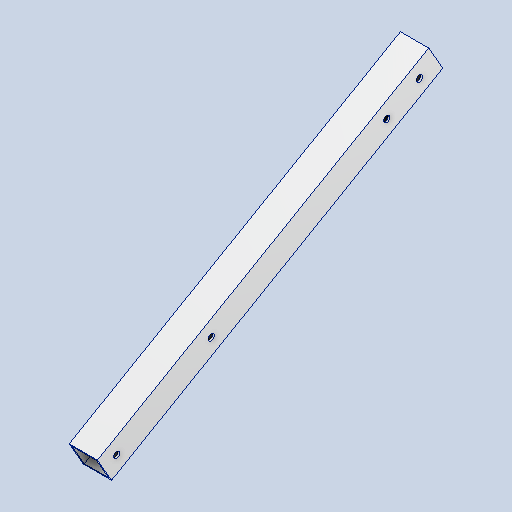
# Autodesk Inventor part: hand-grab-v3-ASP_1
Saved by Autodesk Inventor 2025.1 (Build 291241000, 241)
## iProperties
Created: 2024-11-30
Part Number: hand-grab-v3-ASP_1
Material: アルミニウム 6061
Document SubType Name: Modeling
Designer: haruy
Density: 2.7 g/cm^3
Appearance: アルミニウム - フラット
Author: haruy
Autodesk Inventor part; units mm, degrees
ref_plane "YZ Plane" through (0, 0, 0) normal (1, 0, 0) x (0, 1, 0)
ref_plane "XZ Plane" through (0, 0, 0) normal (0, 1, 0) x (-1, 0, 0)
ref_plane "XY Plane" through (0, 0, 0) normal (0, 0, 1) x (1, 0, 0)
sketch "スケッチ1" plane through (0, 0, 0) normal (1, 0, 0) x (0, 1, 0)
  circle A0 centre (71.3451, 9.7822) radius 120
  line L0 (71.3451, 9.7822) -> (-260.1174, 9.7822) construction
  line L1 (138.8451, -107.1313) -> (-63.6549, 9.7822)
  circle A1 centre (71.3451, 9.7822) radius 5
  line L2 (71.3451, 9.7822) -> (138.8451, 126.6956) construction
  line L3 (71.3451, 9.7822) -> (138.8451, -107.1313) construction
  line L4 (71.3451, 9.7822) -> (-63.6549, 9.7822)
  line L5 (88.381, 47.2892) -> (83.381, 38.629) construction
  line L6 (83.381, 38.629) -> (86.8451, 36.629) construction
  line L7 (86.8451, 36.629) -> (91.8451, 45.2892) construction
  line L8 (91.8451, 45.2892) -> (88.381, 47.2892)
  line L9 (91.8451, 45.2892) -> (86.8451, 36.629) construction
  line L10 (86.8451, 36.629) -> (90.3092, 34.629) construction
  line L11 (90.3092, 34.629) -> (95.3092, 43.2892) construction
  line L12 (95.3092, 43.2892) -> (91.8451, 45.2892)
  line L13 (85.881, 42.9591) -> (92.8092, 38.9591) construction
  circle A2 centre (71.3451, 9.7822) radius 2.65 construction
  line L14 (88.1645, 47.4142) -> (81.6645, 36.1559) construction
  line L15 (81.6645, 36.1559) -> (77.3344, 38.6559) construction
  line L16 (77.3344, 38.6559) -> (83.8344, 49.9142) construction
  line L17 (83.8344, 49.9142) -> (88.1645, 47.4142)
  line L18 (95.5257, 43.1642) -> (89.0257, 31.9059) construction
  line L19 (89.0257, 31.9059) -> (93.3559, 29.4059) construction
  line L20 (93.3559, 29.4059) -> (99.8559, 40.6642) construction
  line L21 (99.8559, 40.6642) -> (95.5257, 43.1642)
  circle A3 centre (71.3451, 9.7822) radius 28.3207 construction
  line L22 (30.3451, 19.0322) -> (30.3451, 14.0322)
  line L23 (30.3451, 14.0322) -> (43.3451, 14.0322) construction
  line L24 (43.3451, 19.0322) -> (30.3451, 19.0322) construction
  line L25 (43.3451, 14.0322) -> (43.3451, 19.0322)
  line L26 (30.3451, 5.5322) -> (43.3451, 5.5322) construction
  line L27 (30.3451, 0.5322) -> (30.3451, 5.5322)
  line L28 (43.3451, 0.5322) -> (30.3451, 0.5322) construction
  line L29 (43.3451, 5.5322) -> (43.3451, 0.5322)
  line L30 (83.8344, -30.3499) -> (88.1645, -27.8499)
  line L31 (88.1645, -27.8499) -> (81.6645, -16.5915) construction
  line L32 (77.3344, -19.0915) -> (83.8344, -30.3499) construction
  line L33 (81.6645, -16.5915) -> (77.3344, -19.0915) construction
  line L34 (95.5257, -23.5999) -> (89.0257, -12.3415) construction
  line L35 (99.8559, -21.0999) -> (95.5257, -23.5999)
  line L36 (93.3559, -9.8415) -> (99.8559, -21.0999) construction
  line L37 (89.0257, -12.3415) -> (93.3559, -9.8415) construction
  line L38 (77.3344, 38.6559) -> (76.7181, 37.5885)
  line L39 (93.3559, 29.4059) -> (92.7396, 28.3385) construction
  line L40 (43.3451, 19.0322) -> (44.5776, 19.0322)
  line L41 (43.3451, 0.5322) -> (44.5776, 0.5322)
  line L42 (77.3344, -19.0915) -> (73.5386, -12.517) construction
  line L43 (93.3559, -9.8415) -> (92.7396, -8.7742) construction
  line L44 (84.956, 41.3569) -> (74.956, 24.0364) construction
  line L45 (74.956, 24.0364) -> (69.7599, 27.0364) construction
  line L46 (69.7599, 27.0364) -> (79.7599, 44.3569) construction
  line L47 (79.7599, 44.3569) -> (84.956, 41.3569)
  circle A4 centre (74.8579, 29.8666) radius 1.5
  circle A5 centre (79.8579, 38.5268) radius 1.5
  circle A6 centre (86.9823, 22.8666) radius 1.5
  circle A7 centre (91.9823, 31.5268) radius 1.5
  circle A8 centre (42.1951, 16.7822) radius 1.5
  circle A9 centre (52.1951, 16.7822) radius 1.5
  circle A10 centre (52.1951, 2.7822) radius 1.5
  circle A11 centre (42.1951, 2.7822) radius 1.5
  circle A12 centre (79.8579, -18.9625) radius 1.5
  circle A13 centre (74.8579, -10.3022) radius 1.5
  circle A14 centre (86.9823, -3.3022) radius 1.5
  circle A15 centre (91.9823, -11.9625) radius 1.5
  line L48 (72.3579, 25.5364) -> (84.956, 41.3569) construction
  circle A16 centre (71.3451, 9.7822) radius 34.3835
  line L49 (63.3451, 56.7822) -> (-116.6549, 56.7822) construction
  line L50 (-116.6549, 56.7822) -> (-116.6549, 41.7822)
  line L51 (-116.6549, 41.7822) -> (63.3451, 41.7822) construction
  line L52 (63.3451, 41.7822) -> (63.3451, 56.7822) construction
  circle A17 centre (53.3451, 49.2822) radius 1.5 construction
  circle A18 centre (43.3451, 49.2822) radius 1.5 construction
  line L53 (36.9617, 56.7822) -> (36.9617, 9.7822) construction
  line L54 (63.3451, 56.7822) -> (90.6652, 38.2244) construction
  line L55 (36.9617, -37.2178) -> (36.9617, 9.7822) construction
  line L56 (63.3451, -37.2178) -> (90.6652, -18.66) construction
  line L57 (63.3451, -37.2178) -> (-116.6549, -37.2178) construction
  line L58 (-116.6549, -22.2178) -> (63.3451, -22.2178) construction
  circle A19 centre (43.3451, -29.7178) radius 1.5 construction
  circle A20 centre (53.3451, -29.7178) radius 1.5 construction
  line L59 (71.3451, 9.7822) -> (54.1534, 39.5591)
  line L60 (62.8136, 44.5591) -> (45.4931, 34.5591)
  line L61 (45.4931, 34.5591) -> (50.4931, 25.8989)
  line L62 (50.4931, 25.8989) -> (67.8136, 35.8989)
  line L63 (67.8136, 35.8989) -> (62.8136, 44.5591)
  circle A21 centre (60.9835, 37.729) radius 1.5
  circle A22 centre (52.3233, 32.729) radius 1.5
  circle A23 centre (52.3233, -13.1647) radius 1.5
  circle A24 centre (60.9835, -18.1647) radius 1.5
  circle A25 centre (100.7286, 4.7822) radius 1.5
  circle A26 centre (100.7286, 14.7822) radius 1.5
  circle A27 centre (71.3451, 9.7822) radius 193.5
  line L64 (-121.5196, 25.4487) -> (154.2099, 184.6412)
  line L65 (71.3451, 9.7822) -> (11.3451, 113.7052)
  line L66 (71.3451, 9.7822) -> (71.3451, 203.2822)
  line L67 (124.6464, 17.4617) -> (23.1464, 193.2648)
  line L68 (23.1464, 193.2648) -> (10.156, 185.7648)
  line L69 (10.156, 185.7648) -> (111.656, 9.9617)
  line L70 (111.656, 9.9617) -> (124.6464, 17.4617)
  circle A28 centre (49.4012, 132.7902) radius 1.5
  circle A29 centre (20.4012, 183.0196) radius 1.5
  circle A30 centre (62.2784, 25.4862) radius 1.5
  circle A31 centre (71.3451, 9.7822) radius 12.5
  circle A32 centre (62.2784, -5.9219) radius 1.5
  circle A33 centre (89.4786, 9.7822) radius 1.5
  circle A34 centre (113.1512, 22.3719) radius 1.5
  circle A35 centre (103.1512, 39.6924) radius 1.5
  circle A36 centre (71.3451, 9.7822) radius 24.3835
  line L71 (124.6464, 17.4617) -> (93.4246, -0.5642)
  line L72 (104.6464, 52.1027) -> (73.4246, 34.0768)
  line L73 (18.0439, 2.1027) -> (49.2656, 20.1286)
  circle A37 centre (29.539, -2.8076) radius 1.5
  circle A38 centre (39.539, -20.1281) radius 1.5
  line L74 (38.0439, -32.5383) -> (-63.4561, 143.2648)
  line L75 (51.0342, -25.0383) -> (38.0439, -32.5383)
  line L76 (38.0439, -32.5383) -> (69.2656, -14.5125)
  point P0 (0, 0)
  point P1 (90.9669, 45.7962)
  point P2 (92.3451, 45.0005)
  point P3 (91.656, 44.6027)
  dimension "d4" = 3
  dimension "d5" = 3
  dimension "d6" = 10
  dimension "d7" = 10
  dimension "d8" = 7.5
  dimension "d9" = 7.5
  dimension "d10" = 60
  dimension "d11" = 10
  dimension "d12" = 10
  dimension "d13" = 10
  dimension "d14" = 3
  dimension "d15" = 5
  dimension "d16" = 5
  dimension "d17" = 360
  dimension "d18" = 387
  dimension "d19" = 110
  dimension "d20" = 60
  dimension "d21" = 15
  dimension "d22" = 73
  dimension "d23" = 3
  dimension "d24" = 3
  dimension "d25" = 7.5
  dimension "d26" = 7.5
  dimension "d27" = 7.5
  dimension "d28" = 7.5
  dimension "d29" = 3
  dimension "d30" = 25
  dimension "d31" = 6.25
  dimension "d32" = 360
  dimension "d33" = 20
  dimension "d34" = 3
  dimension "d35" = 3
  dimension "d36" = 10
  dimension "d37" = 7.5
  dimension "d38" = 7.5
  dimension "d39" = 20
  dimension "d40" = 35
  dimension "d41" = 10
  constraints: 154 end point, 38 centre point, 17 symmetric about line, 8 point on circle, 8 point on line, 6 parallel, 4 perpendicular, 3 coincident, 3 tangent, 1 vertical, 28 other
  measures "d4" diameter of A17
  measures "d5" diameter of A18
  measures "d6" distance from line of A17.centre L52
  measures "d7" distance of A18.centre A17.centre
  measures "d8" distance from line of A17.centre L49
  measures "d9" distance from line of L49 A18.centre
  measures "d11" distance between parallel lines of L60 L62
  measures "d12" distance between parallel lines of L63 L59
  measures "d13" distance between parallel lines of L59 L61
  measures "d14" diameter of A21
  measures "d15" distance from line of L59 A21.centre
  measures "d16" distance from line of A21.centre L60
  measures "d18" diameter of A27
  measures "d19" distance from line of L64 A3.centre
  measures "d21" distance of L68.end L67.end
  measures "d22" distance between parallel lines of L64 L68
  measures "d23" diameter of A28
  measures "d24" diameter of A29
  measures "d25" distance from line of A28.centre L64
  measures "d26" distance from line of A28.centre L69
  measures "d27" distance from line of A29.centre L68
  measures "d28" distance from line of A29.centre L67
  measures "d29" diameter of A30
  measures "d30" diameter of A31
  measures "d31" distance from line of A30.centre L62
  measures "d33" distance from line of L70 point (71.345, 9.782)
  measures "d34" diameter of A34
  measures "d35" diameter of A35
  measures "d36" distance from line of A34.centre L70
  measures "d37" distance from line of L67 A35.centre
  measures "d38" distance from line of L67 A34.centre
  measures "d39" distance of A35.centre A34.centre
  measures "d40" distance from line of L69 point (71.345, 9.782)
  measures "d41" distance from line of L72 A35.centre
extrude "押し出し1" add sketch "スケッチ1" along normal blind 15 contours L67 L66 L69 L64 A0 | A0 L64 L67 | L67 L72 L12 L8 L69 L66 | L64 L69 A0 | A0 L69 L68 L67 L64 | L67 L70 L69 L72 | L8 L12 L72 L69 | A28 | A29 | A34 | A35
shell "シェル1" thickness 1 removed faces 2 at (5, 18.8163, 190.7648) at (5, 115.9861, 12.4617)
hole "穴1" at (0, 138.8451, 126.6956) at (0, -63.6549, 9.7822) at (0, 138.8451, -107.1313) at (0, 20.4012, 183.0196) at (0, 49.4012, 132.7902) at (0, 103.1512, 39.6924) at (0, 113.1512, 22.3719) direction (1, 0, 0) diameter 3.4 end through all
equation "\"d9\" = d8"
